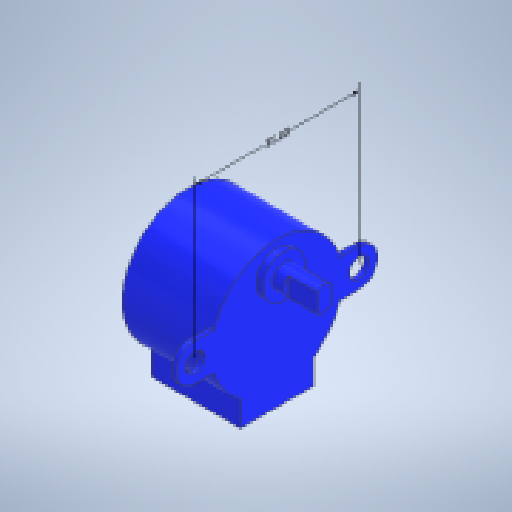
# Autodesk Inventor part: MOTOR
Saved by Autodesk Inventor 2023 (Build 270158000, 158)
## iProperties
Created: 2022-12-02
Part Number: MOTOR
Material: Genérico
Document SubType Name: Modeling
Designer: sergi
Density: 1 g/cm^3
Appearance: Valor por defecto
Author: sergi
Autodesk Inventor part; units mm, degrees
ref_plane "YZ Plane" through (0, 0, 0) normal (1, 0, 0) x (0, 1, 0)
ref_plane "XZ Plane" through (0, 0, 0) normal (0, 1, 0) x (-1, 0, 0)
ref_plane "XY Plane" through (0, 0, 0) normal (0, 0, 1) x (1, 0, 0)
sketch "Boceto1" plane through (0, 0, 0) normal (1, 0, 0) x (0, 1, 0)
  circle A0 centre (0, 0) radius 14
  dimension "d0" = 28
  constraints: 1 centre point, 1 coincident
  measures "d0" diameter of A0
extrude "Extrusión1" add sketch "Boceto1" along normal blind 19
sketch "Boceto2" plane through (19, 0, 0) normal (1, 0, 0) x (0, 0, -1)
  line L0 (0, 0) -> (0, 8)
  circle A0 centre (0, 8) radius 4.5
  dimension "d3" = 8
  dimension "d4" = 9
  constraints: 2 end point, 1 centre point, 1 coincident, 1 vertical
  measures "d3" distance of L0.start L0.end
  measures "d4" diameter of A0
extrude "Extrusión2" add sketch "Boceto2" along normal blind 1.5
sketch "Boceto3" plane through (20.5, 8, 0) normal (1, 0, 0) x (0, 0, -1)
  circle A0 centre (0, 0) radius 2.5
  point P0 (0, -8)
  dimension "d7" = 5
  constraints: 1 centre point
  measures "d7" diameter of A0
extrude "Extrusión3" add sketch "Boceto3" along normal blind 2.5
sketch "Boceto4" plane through (23, 8, 0) normal (1, 0, 0) x (0, 0, -1)
  line L0 (0, 0) -> (-1.5, 0)
  line L1 (-1.5, 0) -> (-1.5, 3)
  line L2 (-1.5, 3) -> (-1.5, -3)
  line L3 (-1.5, -3) -> (1.5, -3)
  line L4 (1.5, -3) -> (1.5, 2.8642)
  circle A0 centre (0, 0) radius 2.5 projected
  point P0 (0, -8)
  point P1 (1.5, 2)
  point P2 (-1.5, 2)
  point P3 (-1.5, -2)
  point P4 (1.5, -2)
  dimension "d10" = 1.5
  dimension "d11" = 3
  constraints: 10 end point, 3 perpendicular, 1 horizontal, 1 point on line
  measures "d10" distance of L0.start L0.end
  measures "d11" distance of L2.end L3.end
extrude "Extrusión4" add sketch "Boceto4" along normal blind 6 contours L1 A0 L4 L2
sketch "Boceto5" plane through (19, 0, 0) normal (1, 0, 0) x (0, 0, -1)
  line L0 (0, 0) -> (17.5, 0)
  circle A0 centre (17.5, 0) radius 2.1
  arc A1 (17.5, -4) -> (17.5, 4) centre (17.5, 0) ccw
  line L1 (17.5, 4) -> (-17.5, 4)
  line L2 (0, 0) -> (0, 18)
  line L3 (-15.4, 0) -> (-17.5, 0)
  circle A2 centre (-17.5, 0) radius 2.1
  arc A3 (-17.5, 4) -> (-17.5, -4) centre (-17.5, 0) ccw
  line L4 (17.5, -4) -> (-17.5, -4)
  dimension "d18" = 4.2
  dimension "d14" = 17.5
  dimension "d15" = 4.2
  dimension "d16" = 8
  dimension "d17" = 17.5
  dimension "d19" = 8
  constraints: 10 end point, 4 coincident, 4 point on circle, 3 centre point, 3 horizontal, 1 horizontal alignment, 1 tangent, 1 vertical, 2 other
  measures "d14" distance of L0.start L0.end
  measures "d15" diameter of A0
  measures "d16" diameter of A1
  measures "d17" distance of L0.start L3.end
  measures "d19" diameter of A3
extrude "Extrusión5" add sketch "Boceto5" against normal blind 1
sketch "Boceto6" plane through (19, 0, 0) normal (1, 0, 0) x (0, 0, -1)
  line L0 (0, 0) -> (0, -17)
  line L1 (0, -17) -> (7.8, -17)
  line L2 (0, -17) -> (-7.8, -17)
  line L3 (-7.8, -17) -> (7.8, -17)
  line L4 (7.8, -17) -> (7.8, -6)
  line L5 (7.8, -6) -> (-7.8, -6)
  line L6 (-7.8, -6) -> (-7.8, -17)
  dimension "d22" = 17
  dimension "d23" = 7.8
  dimension "d25" = 7.8
  constraints: 14 end point, 2 horizontal, 2 parallel, 2 perpendicular, 1 vertical
  measures "d22" distance of L0.start L0.end
  measures "d23" distance of L0.end L1.end
  measures "d25" distance of L0.end L2.end
extrude "Extrusión6" add sketch "Boceto6" against normal blind 19
